Autodesk Fusion 360 part; units mm, degrees
note: some values were not read from the file. Chosen so that the rebuilt part matches the saved one: which bodies a step acts on. Set by a fixed rule: which sketch regions a step uses.
(part 2 of 6)
  spline S18 degree 5 poles (-23.181, 60.8454) (-23.1977, 60.7975) (-23.2312, 60.7019) (-23.2817, 60.5595) (-23.3494, 60.3715) (-23.4348, 60.1397) (-23.5209, 59.9112) (-23.6078, 59.6859) (-23.6954, 59.4641) (-23.7836, 59.2457) (-23.8725, 59.0308) (-23.9619, 58.8195) (-24.0518, 58.6117) (-24.142, 58.4076) (-24.2325, 58.2072) (-24.3233, 58.0106) (-24.4143, 57.8177) (-24.5055, 57.6287) (-24.5967, 57.4436) (-24.6878, 57.2624) (-24.7789, 57.0854) (-24.8696, 56.9125) (-24.96, 56.744) (-25.0498, 56.5799) (-25.1391, 56.4202) (-25.2278, 56.2649) (-25.2983, 56.1442) (-25.3509, 56.0556) (-25.3858, 55.9974) (-25.4032, 55.9685) knots 0 0 0 0 0 0 0.04 0.08 0.12 0.16 0.2 0.24 0.28 0.32 0.36 0.4 0.44 0.48 0.52 0.56 0.6 0.64 0.68 0.72 0.76 0.8 0.84 0.88 0.92 0.96 1 1 1 1 1 1
  arc A18 (-25.4032, 55.9685) -> (-24.3382, 61.9058) centre (-26.2744, 59.1889) ccw
  spline S19 degree 5 poles (-24.3382, 61.9058) (-24.3845, 61.885) (-24.4768, 61.8433) (-24.6143, 61.7806) (-24.7957, 61.6968) (-25.0191, 61.5915) (-25.2393, 61.4858) (-25.4561, 61.3796) (-25.6695, 61.273) (-25.8793, 61.1661) (-26.0857, 61.0588) (-26.2884, 60.9513) (-26.4875, 60.8437) (-26.683, 60.736) (-26.8747, 60.6283) (-27.0627, 60.5207) (-27.2469, 60.4133) (-27.4273, 60.306) (-27.6038, 60.199) (-27.7763, 60.0924) (-27.9447, 59.9863) (-28.109, 59.8809) (-28.2689, 59.7762) (-28.4246, 59.6723) (-28.5759, 59.5695) (-28.7229, 59.4676) (-28.837, 59.3868) (-28.9207, 59.3268) (-28.9756, 59.2869) (-29.0029, 59.267) knots 0 0 0 0 0 0 0.04 0.08 0.12 0.16 0.2 0.24 0.28 0.32 0.36 0.4 0.44 0.48 0.52 0.56 0.6 0.64 0.68 0.72 0.76 0.8 0.84 0.88 0.92 0.96 1 1 1 1 1 1
  arc A19 (-28.7003, 65.566) -> (-29.0029, 59.267) centre (-27.0372, 62.3293) ccw
  spline S20 degree 5 poles (-28.7003, 65.566) (-28.7127, 65.5168) (-28.7378, 65.4186) (-28.7756, 65.2724) (-28.8267, 65.0792) (-28.8915, 64.8408) (-28.9574, 64.6057) (-29.0243, 64.3737) (-29.0923, 64.1451) (-29.1612, 63.9198) (-29.231, 63.698) (-29.3016, 63.4797) (-29.373, 63.2649) (-29.4451, 63.0537) (-29.5179, 62.8462) (-29.5912, 62.6424) (-29.665, 62.4423) (-29.7393, 62.2461) (-29.814, 62.0537) (-29.8891, 61.8653) (-29.9643, 61.681) (-30.0396, 61.5009) (-30.115, 61.3252) (-30.1902, 61.1538) (-30.2652, 60.987) (-30.3401, 60.8245) (-30.3997, 60.6981) (-30.4444, 60.6053) (-30.4741, 60.5443) (-30.489, 60.514) knots 0 0 0 0 0 0 0.04 0.08 0.12 0.16 0.2 0.24 0.28 0.32 0.36 0.4 0.44 0.48 0.52 0.56 0.6 0.64 0.68 0.72 0.76 0.8 0.84 0.88 0.92 0.96 1 1 1 1 1 1
  arc A20 (-30.489, 60.514) -> (-29.9455, 66.5215) centre (-31.6375, 63.6462) ccw
  spline S21 degree 5 poles (-29.9455, 66.5215) (-29.9898, 66.4967) (-30.0781, 66.4471) (-30.2096, 66.3727) (-30.383, 66.2734) (-30.5964, 66.149) (-30.8065, 66.0245) (-31.0132, 65.8999) (-31.2165, 65.7751) (-31.4162, 65.6502) (-31.6125, 65.5254) (-31.8051, 65.4006) (-31.994, 65.2761) (-32.1794, 65.1518) (-32.361, 65.0278) (-32.5389, 64.9042) (-32.713, 64.7811) (-32.8834, 64.6586) (-33.0498, 64.5366) (-33.2124, 64.4154) (-33.3709, 64.295) (-33.5254, 64.1756) (-33.6756, 64.0574) (-33.8217, 63.9404) (-33.9634, 63.8247) (-34.1009, 63.7104) (-34.2076, 63.62) (-34.2857, 63.5529) (-34.337, 63.5084) (-34.3624, 63.4862) knots 0 0 0 0 0 0 0.04 0.08 0.12 0.16 0.2 0.24 0.28 0.32 0.36 0.4 0.44 0.48 0.52 0.56 0.6 0.64 0.68 0.72 0.76 0.8 0.84 0.88 0.92 0.96 1 1 1 1 1 1
  arc A21 (-34.6099, 69.7876) -> (-34.3624, 63.4862) centre (-32.6711, 66.7082) ccw
  spline S22 degree 5 poles (-34.6099, 69.7876) (-34.6181, 69.7374) (-34.6344, 69.6375) (-34.6594, 69.4885) (-34.6934, 69.2916) (-34.7373, 69.0485) (-34.7824, 68.8085) (-34.8289, 68.5716) (-34.8766, 68.3379) (-34.9256, 68.1075) (-34.9758, 67.8804) (-35.0271, 67.6568) (-35.0796, 67.4366) (-35.133, 67.2199) (-35.1874, 67.0069) (-35.2426, 66.7974) (-35.2987, 66.5917) (-35.3557, 66.3897) (-35.4133, 66.1915) (-35.4717, 65.9973) (-35.5306, 65.8072) (-35.5899, 65.6212) (-35.6496, 65.4396) (-35.7096, 65.2623) (-35.7699, 65.0896) (-35.8302, 64.9212) (-35.8787, 64.7901) (-35.9151, 64.6937) (-35.9393, 64.6303) (-35.9515, 64.5989) knots 0 0 0 0 0 0 0.04 0.08 0.12 0.16 0.2 0.24 0.28 0.32 0.36 0.4 0.44 0.48 0.52 0.56 0.6 0.64 0.68 0.72 0.76 0.8 0.84 0.88 0.92 0.96 1 1 1 1 1 1
  arc A22 (-35.9515, 64.5989) -> (-35.9337, 70.6309) centre (-37.3686, 67.6191) ccw
  spline S23 degree 5 poles (-35.9337, 70.6309) (-35.9757, 70.6023) (-36.0593, 70.5452) (-36.1838, 70.4597) (-36.3479, 70.3456) (-36.5497, 70.2031) (-36.7481, 70.0608) (-36.9432, 69.9186) (-37.1348, 69.7765) (-37.3229, 69.6348) (-37.5075, 69.4933) (-37.6885, 69.3522) (-37.8659, 69.2117) (-38.0397, 69.0717) (-38.2098, 68.9324) (-38.3763, 68.7938) (-38.539, 68.656) (-38.698, 68.519) (-38.8532, 68.383) (-39.0046, 68.2481) (-39.1521, 68.1143) (-39.2955, 67.9819) (-39.4349, 67.851) (-39.5701, 67.7217) (-39.7013, 67.5942) (-39.8283, 67.4683) (-39.9267, 67.369) (-39.9987, 67.2953) (-40.0459, 67.2465) (-40.0692, 67.2222) knots 0 0 0 0 0 0 0.04 0.08 0.12 0.16 0.2 0.24 0.28 0.32 0.36 0.4 0.44 0.48 0.52 0.56 0.6 0.64 0.68 0.72 0.76 0.8 0.84 0.88 0.92 0.96 1 1 1 1 1 1
  arc A23 (-40.865, 73.478) -> (-40.0692, 67.2222) centre (-38.6652, 70.5793) ccw
  spline S24 degree 5 poles (-40.865, 73.478) (-40.8688, 73.4274) (-40.8764, 73.3264) (-40.8882, 73.1757) (-40.905, 72.9766) (-40.9275, 72.7306) (-40.9515, 72.4876) (-40.9771, 72.2476) (-41.0043, 72.0106) (-41.0331, 71.7768) (-41.0633, 71.5462) (-41.095, 71.319) (-41.128, 71.095) (-41.1623, 70.8746) (-41.1979, 70.6576) (-41.2347, 70.4441) (-41.2727, 70.2343) (-41.3118, 70.0281) (-41.352, 69.8256) (-41.3931, 69.6271) (-41.4352, 69.4325) (-41.4782, 69.2421) (-41.5218, 69.0559) (-41.5662, 68.8742) (-41.6111, 68.6968) (-41.6566, 68.5238) (-41.6934, 68.389) (-41.7212, 68.2898) (-41.7399, 68.2245) (-41.7493, 68.1921) knots 0 0 0 0 0 0 0.04 0.08 0.12 0.16 0.2 0.24 0.28 0.32 0.36 0.4 0.44 0.48 0.52 0.56 0.6 0.64 0.68 0.72 0.76 0.8 0.84 0.88 0.92 0.96 1 1 1 1 1 1
  arc A24 (-41.7493, 68.1921) -> (-42.2572, 74.2027) centre (-43.4242, 71.0773) ccw
  spline S25 degree 5 poles (-42.2572, 74.2027) (-42.2966, 74.1706) (-42.3749, 74.1065) (-42.4915, 74.0104) (-42.645, 73.8824) (-42.8336, 73.7229) (-43.0189, 73.5638) (-43.2008, 73.4052) (-43.3793, 73.247) (-43.5544, 73.0893) (-43.7259, 72.9323) (-43.894, 72.776) (-44.0584, 72.6205) (-44.2193, 72.4659) (-44.3767, 72.3123) (-44.5304, 72.1597) (-44.6805, 72.0083) (-44.827, 71.858) (-44.9698, 71.709) (-45.1088, 71.5613) (-45.244, 71.4153) (-45.3754, 71.2709) (-45.5029, 71.1283) (-45.6263, 70.9877) (-45.7459, 70.8492) (-45.8614, 70.7127) (-45.9508, 70.6052) (-46.0161, 70.5255) (-46.0588, 70.4728) (-46.08, 70.4466) knots 0 0 0 0 0 0 0.04 0.08 0.12 0.16 0.2 0.24 0.28 0.32 0.36 0.4 0.44 0.48 0.52 0.56 0.6 0.64 0.68 0.72 0.76 0.8 0.84 0.88 0.92 0.96 1 1 1 1 1 1
  arc A25 (-47.418, 76.6092) -> (-46.08, 70.4466) centre (-44.9739, 73.9133) ccw
  spline S26 degree 5 poles (-47.418, 76.6092) (-47.4173, 76.5585) (-47.4161, 76.4572) (-47.4148, 76.3061) (-47.4141, 76.1063) (-47.415, 75.8593) (-47.4178, 75.6151) (-47.4224, 75.3737) (-47.4289, 75.1353) (-47.4371, 74.8999) (-47.4471, 74.6675) (-47.4589, 74.4384) (-47.4722, 74.2124) (-47.4872, 73.9898) (-47.5038, 73.7705) (-47.5218, 73.5547) (-47.5414, 73.3423) (-47.5624, 73.1335) (-47.5847, 72.9283) (-47.6085, 72.7269) (-47.6334, 72.5294) (-47.6596, 72.336) (-47.6869, 72.1468) (-47.7152, 71.9618) (-47.7445, 71.7812) (-47.7747, 71.6049) (-47.7997, 71.4674) (-47.8188, 71.3661) (-47.8317, 71.2995) (-47.8382, 71.2664) knots 0 0 0 0 0 0 0.04 0.08 0.12 0.16 0.2 0.24 0.28 0.32 0.36 0.4 0.44 0.48 0.52 0.56 0.6 0.64 0.68 0.72 0.76 0.8 0.84 0.88 0.92 0.96 1 1 1 1 1 1
  arc A26 (-47.8382, 71.2664) -> (-48.8681, 77.2099) centre (-49.7582, 73.9947) ccw
  spline S27 degree 5 poles (-48.8681, 77.2099) (-48.9045, 77.1745) (-48.9769, 77.1037) (-49.0847, 76.9978) (-49.2264, 76.857) (-49.4004, 76.6816) (-49.5712, 76.507) (-49.7386, 76.3331) (-49.9026, 76.1599) (-50.0632, 75.9876) (-50.2204, 75.8163) (-50.3742, 75.6459) (-50.5245, 75.4767) (-50.6713, 75.3087) (-50.8147, 75.1419) (-50.9545, 74.9765) (-51.0909, 74.8125) (-51.2237, 74.6501) (-51.3529, 74.4892) (-51.4786, 74.33) (-51.6006, 74.1727) (-51.7188, 74.0174) (-51.8334, 73.8643) (-51.9441, 73.7135) (-52.0511, 73.5651) (-52.1544, 73.419) (-52.234, 73.3042) (-52.2921, 73.2191) (-52.3301, 73.1628) (-52.3489, 73.1348) knots 0 0 0 0 0 0 0.04 0.08 0.12 0.16 0.2 0.24 0.28 0.32 0.36 0.4 0.44 0.48 0.52 0.56 0.6 0.64 0.68 0.72 0.76 0.8 0.84 0.88 0.92 0.96 1 1 1 1 1 1
  arc A27 (-54.2189, 79.1574) -> (-52.3489, 73.1348) centre (-51.5491, 76.6848) ccw
  spline S28 degree 5 poles (-54.2189, 79.1574) (-54.2138, 79.1069) (-54.2037, 79.0061) (-54.1893, 78.8557) (-54.1712, 78.6567) (-54.1506, 78.4106) (-54.1321, 78.167) (-54.1157, 77.9262) (-54.1013, 77.6881) (-54.089, 77.4529) (-54.0787, 77.2206) (-54.0704, 76.9913) (-54.0641, 76.765) (-54.0596, 76.5419) (-54.057, 76.322) (-54.0561, 76.1054) (-54.0571, 75.8922) (-54.0598, 75.6823) (-54.0642, 75.476) (-54.0703, 75.2733) (-54.078, 75.0744) (-54.0872, 74.8794) (-54.0979, 74.6885) (-54.1099, 74.5018) (-54.1234, 74.3193) (-54.1381, 74.1411) (-54.151, 74.0019) (-54.1612, 73.8994) (-54.1682, 73.8319) (-54.1718, 73.7983) knots 0 0 0 0 0 0 0.04 0.08 0.12 0.16 0.2 0.24 0.28 0.32 0.36 0.4 0.44 0.48 0.52 0.56 0.6 0.64 0.68 0.72 0.76 0.8 0.84 0.88 0.92 0.96 1 1 1 1 1 1
  arc A28 (-54.1718, 73.7983) -> (-55.7158, 79.6294) centre (-56.3224, 76.3488) ccw
  spline S29 degree 5 poles (-55.7158, 79.6294) (-55.749, 79.591) (-55.815, 79.5142) (-55.9131, 79.3993) (-56.0421, 79.2466) (-56.2001, 79.0568) (-56.355, 78.8679) (-56.5066, 78.6801) (-56.6549, 78.4933) (-56.7999, 78.3077) (-56.9416, 78.1232) (-57.0799, 77.9401) (-57.2149, 77.7584) (-57.3465, 77.5783) (-57.4748, 77.3997) (-57.5997, 77.2227) (-57.7212, 77.0475) (-57.8394, 76.874) (-57.9541, 76.7025) (-58.0654, 76.533) (-58.1732, 76.3656) (-58.2775, 76.2006) (-58.3782, 76.0381) (-58.4754, 75.8782) (-58.5691, 75.721) (-58.6592, 75.5666) (-58.7285, 75.4452) (-58.779, 75.3553) (-58.8119, 75.296) (-58.8282, 75.2665) knots 0 0 0 0 0 0 0.04 0.08 0.12 0.16 0.2 0.24 0.28 0.32 0.36 0.4 0.44 0.48 0.52 0.56 0.6 0.64 0.68 0.72 0.76 0.8 0.84 0.88 0.92 0.96 1 1 1 1 1 1
  arc A29 (-61.216, 81.1032) -> (-58.8282, 75.2665) centre (-58.3409, 78.8726) ccw
  spline S30 degree 5 poles (-61.216, 81.1032) (-61.2065, 81.0533) (-61.1877, 80.9538) (-61.1602, 80.8052) (-61.1249, 80.6086) (-61.0829, 80.3651) (-61.0432, 80.1241) (-61.0059, 79.8857) (-60.9708, 79.6497) (-60.938, 79.4165) (-60.9076, 79.1859) (-60.8793, 78.9582) (-60.8533, 78.7334) (-60.8294, 78.5115) (-60.8076, 78.2927) (-60.7879, 78.077) (-60.7703, 77.8644) (-60.7547, 77.6552) (-60.7411, 77.4492) (-60.7295, 77.2468) (-60.7198, 77.048) (-60.7119, 76.8529) (-60.7059, 76.6618) (-60.7017, 76.4747) (-60.6992, 76.2918) (-60.6984, 76.113) (-60.699, 75.9732) (-60.7003, 75.8702) (-60.7014, 75.8023) (-60.7021, 75.7686) knots 0 0 0 0 0 0 0.04 0.08 0.12 0.16 0.2 0.24 0.28 0.32 0.36 0.4 0.44 0.48 0.52 0.56 0.6 0.64 0.68 0.72 0.76 0.8 0.84 0.88 0.92 0.96 1 1 1 1 1 1
  arc A30 (-60.7021, 75.7686) -> (-62.7484, 81.4429) centre (-63.0667, 78.1219) ccw
  spline S31 degree 5 poles (-62.7484, 81.4429) (-62.7781, 81.4017) (-62.8372, 81.3194) (-62.9249, 81.1964) (-63.04, 81.0331) (-63.1809, 80.8302) (-63.3187, 80.6286) (-63.4534, 80.4283) (-63.5849, 80.2293) (-63.7132, 80.0317) (-63.8382, 79.8356) (-63.9601, 79.6412) (-64.0787, 79.4484) (-64.1941, 79.2574) (-64.3063, 79.0683) (-64.4153, 78.8812) (-64.5211, 78.696) (-64.6237, 78.5129) (-64.723, 78.332) (-64.8191, 78.1534) (-64.912, 77.9773) (-65.0015, 77.8039) (-65.0877, 77.6332) (-65.1706, 77.4655) (-65.2502, 77.3007) (-65.3265, 77.139) (-65.385, 77.012) (-65.4274, 76.9181) (-65.455, 76.8561) (-65.4687, 76.8253) knots 0 0 0 0 0 0 0.04 0.08 0.12 0.16 0.2 0.24 0.28 0.32 0.36 0.4 0.44 0.48 0.52 0.56 0.6 0.64 0.68 0.72 0.76 0.8 0.84 0.88 0.92 0.96 1 1 1 1 1 1
  arc A31 (-68.3561, 82.4317) -> (-65.4687, 76.8253) centre (-65.2975, 80.4602) ccw
  spline S32 degree 5 poles (-68.3561, 82.4317) (-68.3423, 82.3828) (-68.3149, 82.2853) (-68.2745, 82.1397) (-68.2222, 81.9469) (-68.1592, 81.708) (-68.0987, 81.4714) (-68.0406, 81.2371) (-67.9851, 81.0051) (-67.9322, 80.7756) (-67.8817, 80.5486) (-67.8337, 80.3242) (-67.7882, 80.1025) (-67.745, 79.8836) (-67.7043, 79.6675) (-67.6659, 79.4543) (-67.6298, 79.2441) (-67.596, 79.037) (-67.5645, 78.8331) (-67.5353, 78.6324) (-67.5083, 78.4351) (-67.4835, 78.2415) (-67.4609, 78.0517) (-67.4404, 77.8657) (-67.4219, 77.6836) (-67.4055, 77.5056) (-67.394, 77.3663) (-67.3862, 77.2635) (-67.3814, 77.1958) (-67.3792, 77.1622) knots 0 0 0 0 0 0 0.04 0.08 0.12 0.16 0.2 0.24 0.28 0.32 0.36 0.4 0.44 0.48 0.52 0.56 0.6 0.64 0.68 0.72 0.76 0.8 0.84 0.88 0.92 0.96 1 1 1 1 1 1
  arc A32 (-67.3792, 77.1622) -> (-69.9122, 82.6366) centre (-69.9399, 79.3005) ccw
  spline S33 degree 5 poles (-69.9122, 82.6366) (-69.9382, 82.5929) (-69.9899, 82.5058) (-70.0666, 82.3757) (-70.1671, 82.2029) (-70.2898, 81.9885) (-70.4095, 81.7757) (-70.5261, 81.5643) (-70.6398, 81.3546) (-70.7504, 81.1466) (-70.8578, 80.9404) (-70.9623, 80.7361) (-71.0637, 80.5337) (-71.162, 80.3334) (-71.2573, 80.1352) (-71.3496, 79.9393) (-71.4388, 79.7456) (-71.5251, 79.5543) (-71.6083, 79.3654) (-71.6884, 79.1791) (-71.7655, 78.9956) (-71.8396, 78.815) (-71.9106, 78.6375) (-71.9786, 78.4631) (-72.0435, 78.2921) (-72.1054, 78.1243) (-72.1526, 77.9927) (-72.1867, 77.8955) (-72.2088, 77.8314) (-72.2198, 77.7994) knots 0 0 0 0 0 0 0.04 0.08 0.12 0.16 0.2 0.24 0.28 0.32 0.36 0.4 0.44 0.48 0.52 0.56 0.6 0.64 0.68 0.72 0.76 0.8 0.84 0.88 0.92 0.96 1 1 1 1 1 1
  arc A33 (-75.5848, 83.1328) -> (-72.2198, 77.7994) centre (-72.366, 81.4354) ccw
  spline S34 degree 5 poles (-75.5848, 83.1328) (-75.5668, 83.0854) (-75.531, 82.9906) (-75.4781, 82.8491) (-75.4091, 82.6616) (-75.3256, 82.4291) (-75.2446, 82.1987) (-75.1664, 81.9703) (-75.0909, 81.7441) (-75.0182, 81.52) (-74.9481, 81.2983) (-74.8807, 81.0789) (-74.816, 80.862) (-74.754, 80.6477) (-74.6945, 80.436) (-74.6377, 80.227) (-74.5834, 80.0207) (-74.5317, 79.8173) (-74.4826, 79.6169) (-74.436, 79.4195) (-74.3919, 79.2254) (-74.3503, 79.0347) (-74.3112, 78.8475) (-74.2746, 78.664) (-74.2404, 78.4843) (-74.2085, 78.3083) (-74.1849, 78.1705) (-74.1682, 78.0689) (-74.1575, 78.0018) (-74.1523, 77.9685) knots 0 0 0 0 0 0 0.04 0.08 0.12 0.16 0.2 0.24 0.28 0.32 0.36 0.4 0.44 0.48 0.52 0.56 0.6 0.64 0.68 0.72 0.76 0.8 0.84 0.88 0.92 0.96 1 1 1 1 1 1
  arc A34 (-74.1523, 77.9685) -> (-77.1529, 83.2013) centre (-76.8897, 79.8755) ccw
  spline S35 degree 5 poles (-77.1529, 83.2013) (-77.175, 83.1556) (-77.2189, 83.0643) (-77.2839, 82.9279) (-77.369, 82.7471) (-77.4725, 82.5228) (-77.5732, 82.3003) (-77.671, 82.0797) (-77.7659, 81.8609) (-77.8579, 81.644) (-77.9471, 81.4292) (-78.0333, 81.2166) (-78.1166, 81.0061) (-78.1971, 80.798) (-78.2748, 80.5923) (-78.3497, 80.389) (-78.4217, 80.1883) (-78.4909, 79.9902) (-78.5574, 79.7948) (-78.621, 79.6022) (-78.6818, 79.4127) (-78.7398, 79.2263) (-78.7951, 79.0433) (-78.8476, 78.8637) (-78.8974, 78.6876) (-78.9445, 78.5151) (-78.98, 78.3799) (-79.0055, 78.2801) (-79.0219, 78.2142) (-79.03, 78.1815) knots 0 0 0 0 0 0 0.04 0.08 0.12 0.16 0.2 0.24 0.28 0.32 0.36 0.4 0.44 0.48 0.52 0.56 0.6 0.64 0.68 0.72 0.76 0.8 0.84 0.88 0.92 0.96 1 1 1 1 1 1
  arc A35 (-82.8471, 83.2013) -> (-79.03, 78.1815) centre (-79.4926, 81.7909) ccw
  spline S36 degree 5 poles (-82.8471, 83.2013) (-82.825, 83.1556) (-82.7811, 83.0643) (-82.7161, 82.9279) (-82.631, 82.7471) (-82.5275, 82.5228) (-82.4268, 82.3003) (-82.329, 82.0797) (-82.2341, 81.8609) (-82.1421, 81.644) (-82.0529, 81.4292) (-81.9667, 81.2166) (-81.8834, 81.0061) (-81.8029, 80.798) (-81.7252, 80.5923) (-81.6503, 80.389) (-81.5783, 80.1883) (-81.5091, 79.9902) (-81.4426, 79.7948) (-81.379, 79.6022) (-81.3182, 79.4127) (-81.2602, 79.2263) (-81.2049, 79.0433) (-81.1524, 78.8637) (-81.1026, 78.6876) (-81.0555, 78.5151) (-81.02, 78.3799) (-80.9945, 78.2801) (-80.9781, 78.2142) (-80.97, 78.1815) knots 0 0 0 0 0 0 0.04 0.08 0.12 0.16 0.2 0.24 0.28 0.32 0.36 0.4 0.44 0.48 0.52 0.56 0.6 0.64 0.68 0.72 0.76 0.8 0.84 0.88 0.92 0.96 1 1 1 1 1 1
  arc A36 (-80.97, 78.1815) -> (-84.4152, 83.1328) centre (-83.8631, 79.8427) ccw
  spline S37 degree 5 poles (-84.4152, 83.1328) (-84.4332, 83.0854) (-84.469, 82.9906) (-84.5219, 82.8491) (-84.5909, 82.6616) (-84.6744, 82.4291) (-84.7554, 82.1987) (-84.8336, 81.9703) (-84.9091, 81.7441) (-84.9818, 81.52) (-85.0519, 81.2983) (-85.1193, 81.0789) (-85.184, 80.862) (-85.246, 80.6477) (-85.3055, 80.436) (-85.3623, 80.227) (-85.4166, 80.0207) (-85.4683, 79.8173) (-85.5174, 79.6169) (-85.564, 79.4195) (-85.6081, 79.2254) (-85.6497, 79.0347) (-85.6888, 78.8475) (-85.7254, 78.664) (-85.7596, 78.4843) (-85.7915, 78.3083) (-85.8151, 78.1705) (-85.8318, 78.0689) (-85.8425, 78.0018) (-85.8477, 77.9685) knots 0 0 0 0 0 0 0.04 0.08 0.12 0.16 0.2 0.24 0.28 0.32 0.36 0.4 0.44 0.48 0.52 0.56 0.6 0.64 0.68 0.72 0.76 0.8 0.84 0.88 0.92 0.96 1 1 1 1 1 1
  arc A37 (-90.0878, 82.6366) -> (-85.8477, 77.9685) centre (-86.6231, 81.5239) ccw
  spline S38 degree 5 poles (-90.0878, 82.6366) (-90.0618, 82.5929) (-90.0101, 82.5058) (-89.9334, 82.3757) (-89.8329, 82.2029) (-89.7102, 81.9885) (-89.5905, 81.7757) (-89.4739, 81.5643) (-89.3602, 81.3546) (-89.2496, 81.1466) (-89.1422, 80.9404) (-89.0377, 80.7361) (-88.9363, 80.5337) (-88.838, 80.3334) (-88.7427, 80.1352) (-88.6504, 79.9393) (-88.5612, 79.7456) (-88.4749, 79.5543) (-88.3917, 79.3654) (-88.3116, 79.1791) (-88.2345, 78.9956) (-88.1604, 78.815) (-88.0894, 78.6375) (-88.0214, 78.4631) (-87.9565, 78.2921) (-87.8946, 78.1243) (-87.8474, 77.9927) (-87.8133, 77.8955) (-87.7912, 77.8314) (-87.7802, 77.7994) knots 0 0 0 0 0 0 0.04 0.08 0.12 0.16 0.2 0.24 0.28 0.32 0.36 0.4 0.44 0.48 0.52 0.56 0.6 0.64 0.68 0.72 0.76 0.8 0.84 0.88 0.92 0.96 1 1 1 1 1 1
  arc A38 (-87.7802, 77.7994) -> (-91.6439, 82.4317) centre (-90.8072, 79.2021) ccw
  spline S39 degree 5 poles (-91.6439, 82.4317) (-91.6577, 82.3828) (-91.6851, 82.2853) (-91.7255, 82.1397) (-91.7778, 81.9469) (-91.8408, 81.708) (-91.9013, 81.4714) (-91.9594, 81.2371) (-92.0149, 81.0051) (-92.0678, 80.7756) (-92.1183, 80.5486) (-92.1663, 80.3242) (-92.2118, 80.1025) (-92.255, 79.8836) (-92.2957, 79.6675) (-92.3341, 79.4543) (-92.3702, 79.2441) (-92.404, 79.037) (-92.4355, 78.8331) (-92.4647, 78.6324) (-92.4917, 78.4351) (-92.5165, 78.2415) (-92.5391, 78.0517) (-92.5596, 77.8657) (-92.5781, 77.6836) (-92.5945, 77.5056) (-92.606, 77.3663) (-92.6138, 77.2635) (-92.6186, 77.1958) (-92.6208, 77.1622) knots 0 0 0 0 0 0 0.04 0.08 0.12 0.16 0.2 0.24 0.28 0.32 0.36 0.4 0.44 0.48 0.52 0.56 0.6 0.64 0.68 0.72 0.76 0.8 0.84 0.88 0.92 0.96 1 1 1 1 1 1
  arc A39 (-97.2516, 81.4429) -> (-92.6208, 77.1622) centre (-93.7032, 80.6364) ccw
  spline S40 degree 5 poles (-97.2516, 81.4429) (-97.2219, 81.4017) (-97.1628, 81.3194) (-97.0751, 81.1964) (-96.96, 81.0331) (-96.8191, 80.8302) (-96.6813, 80.6286) (-96.5466, 80.4283) (-96.4151, 80.2293) (-96.2868, 80.0317) (-96.1618, 79.8356) (-96.0399, 79.6412) (-95.9213, 79.4484) (-95.8059, 79.2574) (-95.6937, 79.0683) (-95.5847, 78.8812) (-95.4789, 78.696) (-95.3763, 78.5129) (-95.277, 78.332) (-95.1809, 78.1534) (-95.088, 77.9773) (-94.9985, 77.8039) (-94.9123, 77.6332) (-94.8294, 77.4655) (-94.7498, 77.3007) (-94.6735, 77.139) (-94.615, 77.012) (-94.5726, 76.9181) (-94.545, 76.8561) (-94.5313, 76.8253) knots 0 0 0 0 0 0 0.04 0.08 0.12 0.16 0.2 0.24 0.28 0.32 0.36 0.4 0.44 0.48 0.52 0.56 0.6 0.64 0.68 0.72 0.76 0.8 0.84 0.88 0.92 0.96 1 1 1 1 1 1
  arc A40 (-94.5313, 76.8253) -> (-98.784, 81.1032) centre (-97.669, 77.9589) ccw
  spline S41 degree 5 poles (-98.784, 81.1032) (-98.7935, 81.0533) (-98.8123, 80.9538) (-98.8398, 80.8052) (-98.8751, 80.6086) (-98.9171, 80.3651) (-98.9568, 80.1241) (-98.9941, 79.8857) (-99.0292, 79.6497) (-99.062, 79.4165) (-99.0924, 79.1859) (-99.1207, 78.9582) (-99.1467, 78.7334) (-99.1706, 78.5115) (-99.1924, 78.2927) (-99.2121, 78.077) (-99.2297, 77.8644) (-99.2453, 77.6552) (-99.2589, 77.4492) (-99.2705, 77.2468) (-99.2802, 77.048) (-99.2881, 76.8529) (-99.2941, 76.6618) (-99.2983, 76.4747) (-99.3008, 76.2918) (-99.3016, 76.113) (-99.301, 75.9732) (-99.2997, 75.8702) (-99.2986, 75.8023) (-99.2979, 75.7686) knots 0 0 0 0 0 0 0.04 0.08 0.12 0.16 0.2 0.24 0.28 0.32 0.36 0.4 0.44 0.48 0.52 0.56 0.6 0.64 0.68 0.72 0.76 0.8 0.84 0.88 0.92 0.96 1 1 1 1 1 1
  arc A41 (-104.2842, 79.6294) -> (-99.2979, 75.7686) centre (-100.679, 79.1352) ccw
  spline S42 degree 5 poles (-104.2842, 79.6294) (-104.251, 79.591) (-104.185, 79.5142) (-104.0869, 79.3993) (-103.9579, 79.2466) (-103.7999, 79.0568) (-103.645, 78.8679) (-103.4934, 78.6801) (-103.3451, 78.4933) (-103.2001, 78.3077) (-103.0584, 78.1232) (-102.9201, 77.9401) (-102.7851, 77.7584) (-102.6535, 77.5783) (-102.5252, 77.3997) (-102.4003, 77.2227) (-102.2788, 77.0475) (-102.1606, 76.874) (-102.0459, 76.7025) (-101.9346, 76.533) (-101.8268, 76.3656) (-101.7225, 76.2006) (-101.6218, 76.0381) (-101.5246, 75.8782) (-101.4309, 75.721) (-101.3408, 75.5666) (-101.2715, 75.4452) (-101.221, 75.3553) (-101.1881, 75.296) (-101.1718, 75.2665) knots 0 0 0 0 0 0 0.04 0.08 0.12 0.16 0.2 0.24 0.28 0.32 0.36 0.4 0.44 0.48 0.52 0.56 0.6 0.64 0.68 0.72 0.76 0.8 0.84 0.88 0.92 0.96 1 1 1 1 1 1
  arc A42 (-101.1718, 75.2665) -> (-105.7811, 79.1574) centre (-104.3963, 76.1222) ccw
  spline S43 degree 5 poles (-105.7811, 79.1574) (-105.7862, 79.1069) (-105.7963, 79.0061) (-105.8107, 78.8557) (-105.8288, 78.6567) (-105.8494, 78.4106) (-105.8679, 78.167) (-105.8843, 77.9262) (-105.8987, 77.6881) (-105.911, 77.4529) (-105.9213, 77.2206) (-105.9296, 76.9913) (-105.9359, 76.765) (-105.9404, 76.5419) (-105.943, 76.322) (-105.9439, 76.1054) (-105.9429, 75.8922) (-105.9402, 75.6823) (-105.9358, 75.476) (-105.9297, 75.2733) (-105.922, 75.0744) (-105.9128, 74.8794) (-105.9021, 74.6885) (-105.8901, 74.5018) (-105.8766, 74.3193) (-105.8619, 74.1411) (-105.849, 74.0019) (-105.8388, 73.8994) (-105.8318, 73.8319) (-105.8282, 73.7983) knots 0 0 0 0 0 0 0.04 0.08 0.12 0.16 0.2 0.24 0.28 0.32 0.36 0.4 0.44 0.48 0.52 0.56 0.6 0.64 0.68 0.72 0.76 0.8 0.84 0.88 0.92 0.96 1 1 1 1 1 1
  arc A43 (-111.1319, 77.2099) -> (-105.8282, 73.7983) centre (-107.4974, 77.0318) ccw
  spline S44 degree 5 poles (-111.1319, 77.2099) (-111.0955, 77.1745) (-111.0231, 77.1037) (-110.9153, 76.9978) (-110.7736, 76.857) (-110.5996, 76.6816) (-110.4288, 76.507) (-110.2614, 76.3331) (-110.0974, 76.1599) (-109.9368, 75.9876) (-109.7796, 75.8163) (-109.6258, 75.6459) (-109.4755, 75.4767) (-109.3287, 75.3087) (-109.1853, 75.1419) (-109.0455, 74.9765) (-108.9091, 74.8125) (-108.7763, 74.6501) (-108.6471, 74.4892) (-108.5214, 74.33) (-108.3994, 74.1727) (-108.2812, 74.0174) (-108.1666, 73.8643) (-108.0559, 73.7135) (-107.9489, 73.5651) (-107.8456, 73.419) (-107.766, 73.3042) (-107.7079, 73.2191) (-107.6699, 73.1628) (-107.6511, 73.1348) knots 0 0 0 0 0 0 0.04 0.08 0.12 0.16 0.2 0.24 0.28 0.32 0.36 0.4 0.44 0.48 0.52 0.56 0.6 0.64 0.68 0.72 0.76 0.8 0.84 0.88 0.92 0.96 1 1 1 1 1 1
  arc A44 (-107.6511, 73.1348) -> (-112.582, 76.6092) centre (-110.938, 73.7063) ccw
  spline S45 degree 5 poles (-112.582, 76.6092) (-112.5827, 76.5585) (-112.5839, 76.4572) (-112.5852, 76.3061) (-112.5859, 76.1063) (-112.585, 75.8593) (-112.5822, 75.6151) (-112.5776, 75.3737) (-112.5711, 75.1353) (-112.5629, 74.8999) (-112.5529, 74.6675) (-112.5411, 74.4384) (-112.5278, 74.2124) (-112.5128, 73.9898) (-112.4962, 73.7705) (-112.4782, 73.5547) (-112.4586, 73.3423) (-112.4376, 73.1335) (-112.4153, 72.9283) (-112.3915, 72.7269) (-112.3666, 72.5294) (-112.3404, 72.336) (-112.3131, 72.1468) (-112.2848, 71.9618) (-112.2555, 71.7812) (-112.2253, 71.6049) (-112.2003, 71.4674) (-112.1812, 71.3661) (-112.1683, 71.2995) (-112.1618, 71.2664) knots 0 0 0 0 0 0 0.04 0.08 0.12 0.16 0.2 0.24 0.28 0.32 0.36 0.4 0.44 0.48 0.52 0.56 0.6 0.64 0.68 0.72 0.76 0.8 0.84 0.88 0.92 0.96 1 1 1 1 1 1
  arc A45 (-117.7428, 74.2027) -> (-112.1618, 71.2664) centre (-114.1065, 74.3421) ccw
  spline S46 degree 5 poles (-117.7428, 74.2027) (-117.7034, 74.1706) (-117.6251, 74.1065) (-117.5085, 74.0104) (-117.355, 73.8824) (-117.1664, 73.7229) (-116.9811, 73.5638) (-116.7992, 73.4052) (-116.6207, 73.247) (-116.4456, 73.0893) (-116.2741, 72.9323) (-116.106, 72.776) (-115.9416, 72.6205) (-115.7807, 72.4659) (-115.6233, 72.3123) (-115.4696, 72.1597) (-115.3195, 72.0083) (-115.173, 71.858) (-115.0302, 71.709) (-114.8912, 71.5613) (-114.756, 71.4153) (-114.6246, 71.2709) (-114.4971, 71.1283) (-114.3737, 70.9877) (-114.2541, 70.8492) (-114.1386, 70.7127) (-114.0492, 70.6052) (-113.9839, 70.5255) (-113.9412, 70.4728) (-113.92, 70.4466) knots 0 0 0 0 0 0 0.04 0.08 0.12 0.16 0.2 0.24 0.28 0.32 0.36 0.4 0.44 0.48 0.52 0.56 0.6 0.64 0.68 0.72 0.76 0.8 0.84 0.88 0.92 0.96 1 1 1 1 1 1
  arc A46 (-113.92, 70.4466) -> (-119.135, 73.478) centre (-117.2442, 70.7294) ccw
  spline S47 degree 5 poles (-119.135, 73.478) (-119.1312, 73.4274) (-119.1236, 73.3264) (-119.1118, 73.1757) (-119.095, 72.9766) (-119.0725, 72.7306) (-119.0485, 72.4876) (-119.0229, 72.2476) (-118.9957, 72.0106) (-118.9669, 71.7768) (-118.9367, 71.5462) (-118.905, 71.319) (-118.872, 71.095) (-118.8377, 70.8746) (-118.8021, 70.6576) (-118.7653, 70.4441) (-118.7273, 70.2343) (-118.6882, 70.0281) (-118.648, 69.8256) (-118.6069, 69.6271) (-118.5648, 69.4325) (-118.5218, 69.2421) (-118.4782, 69.0559) (-118.4338, 68.8742) (-118.3889, 68.6968) (-118.3434, 68.5238) (-118.3066, 68.389) (-118.2788, 68.2898) (-118.2601, 68.2245) (-118.2507, 68.1921) knots 0 0 0 0 0 0 0.04 0.08 0.12 0.16 0.2 0.24 0.28 0.32 0.36 0.4 0.44 0.48 0.52 0.56 0.6 0.64 0.68 0.72 0.76 0.8 0.84 0.88 0.92 0.96 1 1 1 1 1 1
  arc A47 (-124.0663, 70.6309) -> (-118.2507, 68.1921) centre (-120.4561, 71.0867) ccw
  spline S48 degree 5 poles (-124.0663, 70.6309) (-124.0243, 70.6023) (-123.9407, 70.5452) (-123.8162, 70.4597) (-123.6521, 70.3456) (-123.4503, 70.2031) (-123.2519, 70.0608) (-123.0568, 69.9186) (-122.8652, 69.7765) (-122.6771, 69.6348) (-122.4925, 69.4933) (-122.3115, 69.3522) (-122.1341, 69.2117) (-121.9603, 69.0717) (-121.7902, 68.9324) (-121.6237, 68.7938) (-121.461, 68.656) (-121.302, 68.519) (-121.1468, 68.383) (-120.9954, 68.2481) (-120.8479, 68.1143) (-120.7045, 67.9819) (-120.5651, 67.851) (-120.4299, 67.7217) (-120.2987, 67.5942) (-120.1717, 67.4683) (-120.0733, 67.369) (-120.0013, 67.2953) (-119.9541, 67.2465) (-119.9308, 67.2222) knots 0 0 0 0 0 0 0.04 0.08 0.12 0.16 0.2 0.24 0.28 0.32 0.36 0.4 0.44 0.48 0.52 0.56 0.6 0.64 0.68 0.72 0.76 0.8 0.84 0.88 0.92 0.96 1 1 1 1 1 1
  arc A48 (-119.9308, 67.2222) -> (-125.3901, 69.7876) centre (-123.2669, 67.2142) ccw
  spline S49 degree 5 poles (-125.3901, 69.7876) (-125.3819, 69.7374) (-125.3656, 69.6375) (-125.3406, 69.4885) (-125.3066, 69.2916) (-125.2627, 69.0485) (-125.2176, 68.8085) (-125.1711, 68.5716) (-125.1234, 68.3379) (-125.0744, 68.1075) (-125.0242, 67.8804) (-124.9729, 67.6568) (-124.9204, 67.4366) (-124.867, 67.2199) (-124.8126, 67.0069) (-124.7574, 66.7974) (-124.7013, 66.5917) (-124.6443, 66.3897) (-124.5867, 66.1915) (-124.5283, 65.9973) (-124.4694, 65.8072) (-124.4101, 65.6212) (-124.3504, 65.4396) (-124.2904, 65.2623) (-124.2301, 65.0896) (-124.1698, 64.9212) (-124.1213, 64.7901) (-124.0849, 64.6937) (-124.0607, 64.6303) (-124.0485, 64.5989) knots 0 0 0 0 0 0 0.04 0.08 0.12 0.16 0.2 0.24 0.28 0.32 0.36 0.4 0.44 0.48 0.52 0.56 0.6 0.64 0.68 0.72 0.76 0.8 0.84 0.88 0.92 0.96 1 1 1 1 1 1
  arc A49 (-130.0545, 66.5215) -> (-124.0485, 64.5989) centre (-126.4977, 67.2902) ccw
  spline S50 degree 5 poles (-130.0545, 66.5215) (-130.0102, 66.4967) (-129.9219, 66.4471) (-129.7904, 66.3727) (-129.617, 66.2734) (-129.4036, 66.149) (-129.1935, 66.0245) (-128.9868, 65.8999) (-128.7835, 65.7751) (-128.5838, 65.6502) (-128.3875, 65.5254) (-128.1949, 65.4006) (-128.006, 65.2761) (-127.8206, 65.1518) (-127.639, 65.0278) (-127.4611, 64.9042) (-127.287, 64.7811) (-127.1166, 64.6586) (-126.9502, 64.5366) (-126.7876, 64.4154) (-126.6291, 64.295) (-126.4746, 64.1756) (-126.3244, 64.0574) (-126.1783, 63.9404) (-126.0366, 63.8247) (-125.8991, 63.7104) (-125.7924, 63.62) (-125.7143, 63.5529) (-125.663, 63.5084) (-125.6376, 63.4862) knots 0 0 0 0 0 0 0.04 0.08 0.12 0.16 0.2 0.24 0.28 0.32 0.36 0.4 0.44 0.48 0.52 0.56 0.6 0.64 0.68 0.72 0.76 0.8 0.84 0.88 0.92 0.96 1 1 1 1 1 1
  arc A50 (-125.6376, 63.4862) -> (-131.2997, 65.566) centre (-128.9604, 63.1875) ccw
  spline S51 degree 5 poles (-131.2997, 65.566) (-131.2873, 65.5168) (-131.2622, 65.4186) (-131.2244, 65.2724) (-131.1733, 65.0792) (-131.1085, 64.8408) (-131.0426, 64.6057) (-130.9757, 64.3737) (-130.9077, 64.1451) (-130.8388, 63.9198) (-130.769, 63.698) (-130.6984, 63.4797) (-130.627, 63.2649) (-130.5549, 63.0537) (-130.4821, 62.8462) (-130.4088, 62.6424) (-130.335, 62.4423) (-130.2607, 62.2461) (-130.186, 62.0537) (-130.1109, 61.8653) (-130.0357, 61.681) (-129.9604, 61.5009) (-129.885, 61.3252) (-129.8098, 61.1538) (-129.7348, 60.987) (-129.6599, 60.8245) (-129.6003, 60.6981) (-129.5556, 60.6053) (-129.5259, 60.5443) (-129.511, 60.514) knots 0 0 0 0 0 0 0.04 0.08 0.12 0.16 0.2 0.24 0.28 0.32 0.36 0.4 0.44 0.48 0.52 0.56 0.6 0.64 0.68 0.72 0.76 0.8 0.84 0.88 0.92 0.96 1 1 1 1 1 1
  arc A51 (-135.6618, 61.9058) -> (-129.511, 60.514) centre (-132.1855, 62.9816) ccw
  spline S52 degree 5 poles (-135.6618, 61.9058) (-135.6155, 61.885) (-135.5232, 61.8433) (-135.3857, 61.7806) (-135.2043, 61.6968) (-134.9809, 61.5915) (-134.7607, 61.4858) (-134.5439, 61.3796) (-134.3305, 61.273) (-134.1207, 61.1661) (-133.9143, 61.0588) (-133.7116, 60.9513) (-133.5125, 60.8437) (-133.317, 60.736) (-133.1253, 60.6283) (-132.9373, 60.5207) (-132.7531, 60.4133) (-132.5727, 60.306) (-132.3962, 60.199) (-132.2237, 60.0924) (-132.0553, 59.9863) (-131.891, 59.8809) (-131.7311, 59.7762) (-131.5754, 59.6723) (-131.4241, 59.5695) (-131.2771, 59.4676) (-131.163, 59.3868) (-131.0793, 59.3268) (-131.0244, 59.2869) (-130.9971, 59.267) knots 0 0 0 0 0 0 0.04 0.08 0.12 0.16 0.2 0.24 0.28 0.32 0.36 0.4 0.44 0.48 0.52 0.56 0.6 0.64 0.68 0.72 0.76 0.8 0.84 0.88 0.92 0.96 1 1 1 1 1 1
  arc A52 (-130.9971, 59.267) -> (-136.819, 60.8454) centre (-134.2812, 58.6799) ccw
  spline S53 degree 5 poles (-136.819, 60.8454) (-136.8023, 60.7975) (-136.7688, 60.7019) (-136.7183, 60.5595) (-136.6506, 60.3715) (-136.5652, 60.1397) (-136.4791, 59.9112) (-136.3922, 59.6859) (-136.3046, 59.4641) (-136.2164, 59.2457) (-136.1275, 59.0308) (-136.0381, 58.8195) (-135.9482, 58.6117) (-135.858, 58.4076) (-135.7675, 58.2072) (-135.6767, 58.0106) (-135.5857, 57.8177) (-135.4945, 57.6287) (-135.4033, 57.4436) (-135.3122, 57.2624) (-135.2211, 57.0854) (-135.1304, 56.9125) (-135.04, 56.744) (-134.9502, 56.5799) (-134.8609, 56.4202) (-134.7722, 56.2649) (-134.7017, 56.1442) (-134.6491, 56.0556) (-134.6142, 55.9974) (-134.5968, 55.9685) knots 0 0 0 0 0 0 0.04 0.08 0.12 0.16 0.2 0.24 0.28 0.32 0.36 0.4 0.44 0.48 0.52 0.56 0.6 0.64 0.68 0.72 0.76 0.8 0.84 0.88 0.92 0.96 1 1 1 1 1 1
  arc A53 (-140.8454, 56.819) -> (-134.5968, 55.9685) centre (-137.4761, 58.1936) ccw
  spline S54 degree 5 poles (-140.8454, 56.819) (-140.7975, 56.8023) (-140.7019, 56.7688) (-140.5595, 56.7183) (-140.3715, 56.6506) (-140.1397, 56.5652) (-139.9112, 56.4791) (-139.6859, 56.3922) (-139.4641, 56.3046) (-139.2457, 56.2164) (-139.0308, 56.1275) (-138.8195, 56.0381) (-138.6117, 55.9482) (-138.4076, 55.858) (-138.2072, 55.7675) (-138.0106, 55.6767) (-137.8177, 55.5857) (-137.6287, 55.4945) (-137.4436, 55.4033) (-137.2624, 55.3122) (-137.0854, 55.2211) (-136.9125, 55.1304) (-136.744, 55.04) (-136.5799, 54.9502) (-136.4202, 54.8609) (-136.2649, 54.7722) (-136.1442, 54.7017) (-136.0556, 54.6491) (-135.9974, 54.6142) (-135.9685, 54.5968) knots 0 0 0 0 0 0 0.04 0.08 0.12 0.16 0.2 0.24 0.28 0.32 0.36 0.4 0.44 0.48 0.52 0.56 0.6 0.64 0.68 0.72 0.76 0.8 0.84 0.88 0.92 0.96 1 1 1 1 1 1
  arc A54 (-135.9685, 54.5968) -> (-141.9058, 55.6618) centre (-139.1889, 53.7256) ccw
  spline S55 degree 5 poles (-141.9058, 55.6618) (-141.885, 55.6155) (-141.8433, 55.5232) (-141.7806, 55.3857) (-141.6968, 55.2043) (-141.5915, 54.9809) (-141.4858, 54.7607) (-141.3796, 54.5439) (-141.273, 54.3305) (-141.1661, 54.1207) (-141.0588, 53.9143) (-140.9513, 53.7116) (-140.8437, 53.5125) (-140.736, 53.317) (-140.6283, 53.1253) (-140.5207, 52.9373) (-140.4133, 52.7531) (-140.306, 52.5727) (-140.199, 52.3962) (-140.0924, 52.2237) (-139.9863, 52.0553) (-139.8809, 51.891) (-139.7762, 51.7311) (-139.6723, 51.5754) (-139.5695, 51.4241) (-139.4676, 51.2771) (-139.3868, 51.163) (-139.3268, 51.0793) (-139.2869, 51.0244) (-139.267, 50.9971) knots 0 0 0 0 0 0 0.04 0.08 0.12 0.16 0.2 0.24 0.28 0.32 0.36 0.4 0.44 0.48 0.52 0.56 0.6 0.64 0.68 0.72 0.76 0.8 0.84 0.88 0.92 0.96 1 1 1 1 1 1
  arc A55 (-145.566, 51.2997) -> (-139.267, 50.9971) centre (-142.3293, 52.9628) ccw
  spline S56 degree 5 poles (-145.566, 51.2997) (-145.5168, 51.2873) (-145.4186, 51.2622) (-145.2724, 51.2244) (-145.0792, 51.1733) (-144.8408, 51.1085) (-144.6057, 51.0426) (-144.3737, 50.9757) (-144.1451, 50.9077) (-143.9198, 50.8388) (-143.698, 50.769) (-143.4797, 50.6984) (-143.2649, 50.627) (-143.0537, 50.5549) (-142.8462, 50.4821) (-142.6424, 50.4088) (-142.4423, 50.335) (-142.2461, 50.2607) (-142.0537, 50.186) (-141.8653, 50.1109) (-141.681, 50.0357) (-141.5009, 49.9604) (-141.3252, 49.885) (-141.1538, 49.8098) (-140.987, 49.7348) (-140.8245, 49.6599) (-140.6981, 49.6003) (-140.6053, 49.5556) (-140.5443, 49.5259) (-140.514, 49.511) knots 0 0 0 0 0 0 0.04 0.08 0.12 0.16 0.2 0.24 0.28 0.32 0.36 0.4 0.44 0.48 0.52 0.56 0.6 0.64 0.68 0.72 0.76 0.8 0.84 0.88 0.92 0.96 1 1 1 1 1 1
  arc A56 (-140.514, 49.511) -> (-146.5215, 50.0545) centre (-143.6462, 48.3625) ccw
  spline S57 degree 5 poles (-146.5215, 50.0545) (-146.4967, 50.0102) (-146.4471, 49.9219) (-146.3727, 49.7904) (-146.2734, 49.617) (-146.149, 49.4036) (-146.0245, 49.1935) (-145.8999, 48.9868) (-145.7751, 48.7835) (-145.6502, 48.5838) (-145.5254, 48.3875) (-145.4006, 48.1949) (-145.2761, 48.006) (-145.1518, 47.8206) (-145.0278, 47.639) (-144.9042, 47.4611) (-144.7811, 47.287) (-144.6586, 47.1166) (-144.5366, 46.9502) (-144.4154, 46.7876) (-144.295, 46.6291) (-144.1756, 46.4746) (-144.0574, 46.3244) (-143.9404, 46.1783) (-143.8247, 46.0366) (-143.7104, 45.8991) (-143.62, 45.7924) (-143.5529, 45.7143) (-143.5084, 45.663) (-143.4862, 45.6376) knots 0 0 0 0 0 0 0.04 0.08 0.12 0.16 0.2 0.24 0.28 0.32 0.36 0.4 0.44 0.48 0.52 0.56 0.6 0.64 0.68 0.72 0.76 0.8 0.84 0.88 0.92 0.96 1 1 1 1 1 1
  arc A57 (-149.7876, 45.3901) -> (-143.4862, 45.6376) centre (-146.7082, 47.3289) ccw
  spline S58 degree 5 poles (-149.7876, 45.3901) (-149.7374, 45.3819) (-149.6375, 45.3656) (-149.4885, 45.3406) (-149.2916, 45.3066) (-149.0485, 45.2627) (-148.8085, 45.2176) (-148.5716, 45.1711) (-148.3379, 45.1234) (-148.1075, 45.0744) (-147.8804, 45.0242) (-147.6568, 44.9729) (-147.4366, 44.9204) (-147.2199, 44.867) (-147.0069, 44.8126) (-146.7974, 44.7574) (-146.5917, 44.7013) (-146.3897, 44.6443) (-146.1915, 44.5867) (-145.9973, 44.5283) (-145.8072, 44.4694) (-145.6212, 44.4101) (-145.4396, 44.3504) (-145.2623, 44.2904) (-145.0896, 44.2301) (-144.9212, 44.1698) (-144.7901, 44.1213) (-144.6937, 44.0849) (-144.6303, 44.0607) (-144.5989, 44.0485) knots 0 0 0 0 0 0 0.04 0.08 0.12 0.16 0.2 0.24 0.28 0.32 0.36 0.4 0.44 0.48 0.52 0.56 0.6 0.64 0.68 0.72 0.76 0.8 0.84 0.88 0.92 0.96 1 1 1 1 1 1
  arc A58 (-144.5989, 44.0485) -> (-150.6309, 44.0663) centre (-147.6191, 42.6314) ccw
  spline S59 degree 5 poles (-150.6309, 44.0663) (-150.6023, 44.0243) (-150.5452, 43.9407) (-150.4597, 43.8162) (-150.3456, 43.6521) (-150.2031, 43.4503) (-150.0608, 43.2519) (-149.9186, 43.0568) (-149.7765, 42.8652) (-149.6348, 42.6771) (-149.4933, 42.4925) (-149.3522, 42.3115) (-149.2117, 42.1341) (-149.0717, 41.9603) (-148.9324, 41.7902) (-148.7938, 41.6237) (-148.656, 41.461) (-148.519, 41.302) (-148.383, 41.1468) (-148.2481, 40.9954) (-148.1143, 40.8479) (-147.9819, 40.7045) (-147.851, 40.5651) (-147.7217, 40.4299) (-147.5942, 40.2987) (-147.4683, 40.1717) (-147.369, 40.0733) (-147.2953, 40.0013) (-147.2465, 39.9541) (-147.2222, 39.9308) knots 0 0 0 0 0 0 0.04 0.08 0.12 0.16 0.2 0.24 0.28 0.32 0.36 0.4 0.44 0.48 0.52 0.56 0.6 0.64 0.68 0.72 0.76 0.8 0.84 0.88 0.92 0.96 1 1 1 1 1 1
  arc A59 (-153.478, 39.135) -> (-147.2222, 39.9308) centre (-150.5793, 41.3348) ccw
  spline S60 degree 5 poles (-153.478, 39.135) (-153.4274, 39.1312) (-153.3264, 39.1236) (-153.1757, 39.1118) (-152.9766, 39.095) (-152.7306, 39.0725) (-152.4876, 39.0485) (-152.2476, 39.0229) (-152.0106, 38.9957) (-151.7768, 38.9669) (-151.5462, 38.9367) (-151.319, 38.905) (-151.095, 38.872) (-150.8746, 38.8377) (-150.6576, 38.8021) (-150.4441, 38.7653) (-150.2343, 38.7273) (-150.0281, 38.6882) (-149.8256, 38.648) (-149.6271, 38.6069) (-149.4325, 38.5648) (-149.2421, 38.5218) (-149.0559, 38.4782) (-148.8742, 38.4338) (-148.6968, 38.3889) (-148.5238, 38.3434) (-148.389, 38.3066) (-148.2898, 38.2788) (-148.2245, 38.2601) (-148.1921, 38.2507) knots 0 0 0 0 0 0 0.04 0.08 0.12 0.16 0.2 0.24 0.28 0.32 0.36 0.4 0.44 0.48 0.52 0.56 0.6 0.64 0.68 0.72 0.76 0.8 0.84 0.88 0.92 0.96 1 1 1 1 1 1
  arc A60 (-148.1921, 38.2507) -> (-154.2027, 37.7428) centre (-151.0773, 36.5758) ccw